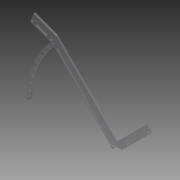
# Autodesk Inventor part: Inner Rail
Saved by Autodesk Inventor 2013 (Build 170138000, 138)
## iProperties
Created: 2013-01-27
Part Number: Inner Rail
Material: Polycarbonate, Clear
Document SubType Name: Modeling
Designer: Andrew Toennies
Density: 1.2 g/cm^3
Mass: 148.156 g
Surface Area: 555.15 cm^2
Volume: 123.463 cm^3
Author: Andrew Toennies
Autodesk Inventor part; units mm, degrees
ref_plane "YZ Plane" through (0, 0, 0) normal (1, 0, 0) x (0, 1, 0)
ref_plane "XZ Plane" through (0, 0, 0) normal (0, 1, 0) x (-1, 0, 0)
ref_plane "XY Plane" through (0, 0, 0) normal (0, 0, 1) x (1, 0, 0)
sketch "Sketch1" plane through (0, 0, 0) normal (0, 0, 1) x (1, 0, 0)
  circle A0 centre (-295.4793, 52.101) radius 1.5875
  circle A1 centre (-281.943, 102.6189) radius 1.5875
  circle A2 centre (-259.8401, 150.0188) radius 1.5875
  circle A3 centre (-229.8421, 192.8604) radius 1.5875
  circle A4 centre (-219.9695, 210.9892) radius 1.5875
  circle A5 centre (-300.1694, 52.928) radius 1.5875
  circle A6 centre (-286.4183, 104.2477) radius 1.5875
  circle A7 centre (-263.9645, 152.4) radius 1.5875
  circle A8 centre (-233.4903, 195.9217) radius 1.5875
  circle A9 centre (-249.6775, 174.8261) radius 1.5875
  circle A10 centre (-276.2426, 128.814) radius 1.5875
  circle A11 centre (-294.4142, 78.888) radius 1.5875
  circle A12 centre (-303.6401, 26.5651) radius 1.5875
  circle A13 centre (-304.7338, 6.35) radius 1.5875
  circle A14 centre (-245.7763, 172.0944) radius 1.5875
  circle A15 centre (-271.9263, 126.8013) radius 1.5875
  circle A16 centre (-289.814, 77.6554) radius 1.5875
  circle A17 centre (-298.8958, 26.15) radius 1.5875
  arc A18 (-220.0163, 220.0163) -> (-311.15, 0) centre (0, 0) ccw
  line L0 (-311.15, 0) -> (0, 0)
  line L1 (0, 0) -> (-220.0163, 220.0163)
  arc A19 (-209.9135, 209.9135) -> (-296.8625, 0) centre (0, 0) ccw
  arc A20 (-220.0163, 220.0163) -> (-311.15, 0) centre (0, 0) ccw
  dimension "d0" = 593.725
  constraints: 21 centre point, 6 point on circle, 4 end point, 2 coincident, 2 point on line, 1 horizontal, 43 other
  measures "d0" diameter of A19
extrude "Extrusion1" add sketch "Sketch1" along normal blind 6.35 contours L1 A19 L0 A18
sketch "Sketch2" plane through (0, 0, 6.35) normal (0, 0, 1) x (1, 0, 0)
  arc A0 (-220.0163, 220.0163) -> (-311.15, 0) centre (0, 0) ccw projected
  line L0 (-311.15, 0) -> (-296.8625, 0) projected
  line L1 (-311.15, 0) -> (-311.15, -6.35)
  line L2 (-311.15, -6.35) -> (-304.8, -6.35)
  line L3 (-304.8, -6.35) -> (-304.8, 0)
  dimension "d3" = 6.35
  dimension "d4" = 6.35
  constraints: 6 end point, 3 perpendicular, 1 point on line, 1 tangent
  measures "d3" distance of L0.start L1.end
  measures "d4" distance of L1.end L2.end
extrude "Extrusion2" add sketch "Sketch2" against normal blind 6.35
sketch "Sketch3" plane through (0, 0, 0) normal (0, 0, -1) x (-1, 0, 0)
  arc A0 (311.15, 0) -> (220.0163, 220.0163) centre (0, 0) ccw projected
  line L0 (311.15, -6.35) -> (311.15, 0) projected
  line L1 (220.0163, 220.0163) -> (177.0122, 220.0163)
  circle A1 centre (281.943, 102.6189) radius 1.5875 projected
  circle A2 centre (263.9645, 152.4) radius 1.5875 projected
  circle A3 centre (276.2426, 128.814) radius 1.5875 projected
  circle A4 centre (245.7763, 172.0944) radius 1.5875 projected
  circle A5 centre (249.6775, 174.8261) radius 1.5875 projected
  circle A6 centre (286.4183, 104.2477) radius 1.5875 projected
  circle A7 centre (295.4793, 52.101) radius 1.5875 projected
  circle A8 centre (259.8401, 150.0188) radius 1.5875 projected
  circle A9 centre (233.4903, 195.9217) radius 1.5875 projected
  circle A10 centre (294.4142, 78.888) radius 1.5875 projected
  circle A11 centre (289.814, 77.6554) radius 1.5875 projected
  circle A12 centre (271.9263, 126.8013) radius 1.5875 projected
  circle A13 centre (300.1694, 52.928) radius 1.5875 projected
  circle A14 centre (219.9695, 210.9892) radius 1.5875 projected
  circle A15 centre (229.8421, 192.8604) radius 1.5875 projected
  arc A16 (311.15, 0) -> (224.8896, 215.0325) centre (0, 0) ccw projected
  line L2 (224.8896, 215.0325) -> (296.2163, 240.9933) projected
  line L3 (296.2163, 240.9933) -> (296.2163, 247.7508) projected
  line L4 (296.2163, 247.7508) -> (220.0163, 220.0163) projected
  line L5 (220.0163, 220.0163) -> (209.9135, 209.9135) projected
  arc A17 (293.5158, 44.45) -> (209.9135, 209.9135) centre (0, 0) ccw projected
  line L6 (293.5158, 44.45) -> (301.625, 44.45) projected
  line L7 (301.625, 44.45) -> (301.625, 0) projected
  line L8 (301.625, 0) -> (304.8, 0) projected
  line L9 (304.8, 0) -> (304.8, -6.35) projected
  line L10 (304.8, -6.35) -> (311.15, -6.35) projected
  line L11 (311.15, -6.35) -> (311.15, 0) projected
  constraints: 2 end point, 1 perpendicular
extrude "Extrusion3" add sketch "Sketch3" against normal blind 6.35 contours A0 L4 L3 L2
sketch "Sketch4" plane through (0, 0, 0) normal (0, 0, -1) x (-1, 0, 0)
  line L0 (209.9135, 209.9135) -> (220.0163, 220.0163) projected
  arc A0 (296.8625, 0) -> (209.9135, 209.9135) centre (0, 0) ccw projected
  arc A1 (311.15, 0) -> (224.8896, 215.0325) centre (0, 0) ccw projected
  line L1 (0, 0) -> (209.9135, 209.9135)
  line L2 (6.35, -6.35) -> (0, -6.35) projected
  line L3 (6.35, 0) -> (6.35, -6.35) projected
  line L4 (0, 0) -> (6.35, 0) projected
  line L5 (0, 0) -> (0, -6.35) projected
  line L6 (0, -6.35) -> (0, 0)
  line L7 (0, -6.35) -> (6.35, -6.35)
  line L8 (6.35, 0) -> (6.35, -6.35)
  line L9 (6.35, 0) -> (213.0645, 206.7145)
  constraints: 10 end point, 4 collinear, 1 parallel, 1 point on circle
extrude "Extrusion4" add sketch "Sketch4" against normal blind 6.35
sketch "Sketch7" plane through (0, 0, 0) normal (0, 0, -1) x (-1, 0, 0)
  line L0 (220.0163, 220.0163) -> (0, 0) projected
  line L1 (296.2163, 247.7508) -> (220.0163, 220.0163) projected
  line L2 (0, 0) -> (220.0163, 220.0163) projected
  line L3 (202.0558, 206.5459) -> (211.036, 215.5261) projected
  line L4 (204.3008, 204.3008) -> (202.0558, 206.5459) projected
  line L5 (213.2811, 213.2811) -> (204.3008, 204.3008) projected
  line L6 (211.036, 215.5261) -> (213.2811, 213.2811) projected
  line L7 (-134.4395, 156.8901) -> (11.2253, 11.2253) projected
  line L8 (8.9803, 13.4704) -> (13.4704, 17.9605) projected
  line L9 (15.7154, 15.7154) -> (13.4704, 17.9605)
  line L10 (13.4704, 17.9605) -> (8.9803, 13.4704)
  line L11 (8.9803, 13.4704) -> (-8.9803, 31.4309)
  line L12 (15.7154, 15.7154) -> (24.6957, 24.6957)
  line L13 (24.6957, 24.6957) -> (22.4506, 26.9408)
  line L14 (22.4506, 26.9408) -> (202.0558, 206.5459)
  line L15 (202.0558, 206.5459) -> (204.3008, 204.3008)
  line L16 (204.3008, 204.3008) -> (213.2811, 213.2811)
  line L17 (213.2811, 213.2811) -> (211.036, 215.5261)
  line L18 (220.0163, 220.0163) -> (216.1966, 226.012)
  line L19 (211.036, 215.5261) -> (218.2689, 222.7591)
  line L20 (218.2689, 222.7591) -> (204.2902, 244.7013)
  line L21 (-8.9803, 31.4309) -> (204.2902, 244.7013)
  line L22 (204.3008, 204.3008) -> (202.0558, 206.5459) projected
  line L23 (211.036, 215.5261) -> (213.2811, 213.2811) projected
  line L24 (202.0558, 206.5459) -> (211.036, 215.5261) projected
  line L25 (213.2811, 213.2811) -> (204.3008, 204.3008) projected
  point P0 (8.9803, 8.9803)
  dimension "d19" = 25.4
  dimension "d20" = 102.5
  constraints: 26 end point, 5 collinear, 4 perpendicular, 2 point on line, 1 parallel
  measures "d19" distance of L8.start L11.end
  measures "d20" angle of L1 L18
extrude "Extrusion7" add sketch "Sketch7" against normal blind 6.35 contours L0 L4 L3 L6 | L19 L3 L14 L13 L0 L9 L8 L7 L21 L20 L18
sketch "Sketch8" plane through (0, 0, 0) normal (0, 0, -1) x (-1, 0, 0)
  line L0 (211.036, 215.5261) -> (218.2689, 222.7591) projected
  line L1 (218.2689, 222.7591) -> (204.2902, 244.7013) projected
  line L2 (296.2163, 247.7508) -> (220.0163, 220.0163) projected
  line L3 (238.4434, 230.102) -> (239.5293, 227.1184) projected
  line L4 (226.5093, 225.7583) -> (238.4434, 230.102) projected
  line L5 (227.5952, 222.7748) -> (226.5093, 225.7583) projected
  line L6 (239.5293, 227.1184) -> (227.5952, 222.7748) projected
  line L7 (220.5423, 223.5865) -> (221.6282, 220.603) projected
  line L8 (290.2492, 245.579) -> (278.3151, 241.2353) projected
  line L9 (289.1633, 248.5625) -> (290.2492, 245.579) projected
  line L10 (277.2292, 244.2188) -> (289.1633, 248.5625) projected
  line L11 (278.3151, 241.2353) -> (277.2292, 244.2188) projected
  line L12 (217.7712, 217.7712) -> (215.5261, 220.0163) projected
  line L13 (218.2689, 222.7591) -> (215.5261, 220.0163)
  line L14 (215.5261, 220.0163) -> (217.7712, 217.7712)
  line L15 (217.7712, 217.7712) -> (220.0163, 220.0163)
  line L16 (221.6282, 220.603) -> (220.0465, 220.0273)
  line L17 (221.6282, 220.603) -> (220.5423, 223.5865)
  line L18 (204.2902, 244.7013) -> (286.443, 274.6025)
  line L19 (295.1304, 250.7343) -> (296.2163, 247.7508) projected
  line L20 (295.1304, 250.7343) -> (286.443, 274.6025)
  line L21 (218.2689, 222.7591) -> (204.2902, 244.7013)
  line L22 (295.1304, 250.7343) -> (289.1633, 248.5625)
  line L23 (289.1633, 248.5625) -> (290.2492, 245.579)
  line L24 (290.2492, 245.579) -> (278.3151, 241.2353)
  line L25 (278.3151, 241.2353) -> (277.2292, 244.2188)
  line L26 (277.2292, 244.2188) -> (238.4434, 230.102)
  line L27 (238.4434, 230.102) -> (239.5293, 227.1184)
  line L28 (239.5293, 227.1184) -> (227.5952, 222.7748)
  line L29 (226.5093, 225.7583) -> (227.5952, 222.7748)
  line L30 (220.5423, 223.5865) -> (226.5093, 225.7583)
  constraints: 34 end point, 10 perpendicular, 5 collinear, 2 point on line
extrude "Extrusion8" add sketch "Sketch8" against normal blind 6.35 contours L0 L1 L18 L20 L22 L10 L26 L4 L30 L7 L2 L15 L12 | L9 L2 L11 L10 | L5 L4 L3 L2
sketch "Sketch11" plane through (0, 0, 0) normal (0, 0, -1) x (-1, 0, 0)
  line L0 (-8.9803, 31.4309) -> (8.9803, 13.4704) projected
  line L1 (296.2163, 240.9933) -> (296.2163, 247.7508) projected
  line L2 (204.3008, 204.3008) -> (24.6957, 24.6957) projected
  line L3 (-8.9803, 31.4309) -> (-33.676, 6.7352)
  line L4 (8.9803, 13.4704) -> (2.2451, 6.7352)
  line L5 (-33.676, 6.7352) -> (2.2451, 6.7352)
  dimension "d35" = 34.925
  constraints: 6 end point, 2 parallel, 1 perpendicular
  measures "d35" distance of L0.start L3.end
extrude "Extrusion11" add sketch "Sketch11" against normal blind 6.35
sketch "Sketch12" plane through (0, 0, 0) normal (0, 0, -1) x (-1, 0, 0)
  line L0 (204.2902, 244.7013) -> (-33.676, 6.7352) projected
  line L1 (204.3008, 204.3008) -> (24.6957, 24.6957) projected
  line L2 (-33.676, 6.7352) -> (-141.439, 114.4983)
  line L3 (-141.439, 114.4983) -> (-123.4785, 132.4588)
  line L4 (-123.4785, 132.4588) -> (-15.7154, 24.6957)
  line L5 (-134.7038, 112.2532) -> (-132.4588, 114.4983)
  line L6 (-132.4588, 114.4983) -> (-123.4785, 105.518)
  line L7 (-123.4785, 105.518) -> (-125.7236, 103.2729)
  line L8 (-125.7236, 103.2729) -> (-134.7038, 112.2532)
  line L9 (-60.6167, 42.6562) -> (-62.8618, 40.4112)
  line L10 (-62.8618, 40.4112) -> (-53.8815, 31.4309)
  line L11 (-53.8815, 31.4309) -> (-51.6365, 33.676)
  line L12 (-51.6365, 33.676) -> (-60.6167, 42.6562)
  dimension "d38" = 152.4
  dimension "d39" = 25.4
  dimension "d40" = 3.175
  dimension "d41" = 12.7
  dimension "d42" = 6.35
  dimension "d43" = 3.175
  dimension "d44" = 3.175
  dimension "d45" = 12.7
  dimension "d46" = 3.175
  dimension "d47" = 3.175
  dimension "d48" = 88.9
  constraints: 22 end point, 8 perpendicular, 2 parallel, 1 point on line
  measures "d38" distance of L0.end L2.end
  measures "d39" distance of L2.end L3.end
  measures "d40" distance of L5.start L5.end
  measures "d41" distance of L5.end L6.end
  measures "d42" distance between parallel lines of L3 L5
  measures "d43" distance between parallel lines of L2 L8
  measures "d44" distance of L9.start L9.end
  measures "d45" distance of L9.end L10.end
  measures "d46" distance of L10.end L11.end
  measures "d47" distance between parallel lines of L2 L10
  measures "d48" distance between parallel lines of L7 L9
extrude "Extrusion12" add sketch "Sketch12" against normal blind 6.35
body "Solid1"
